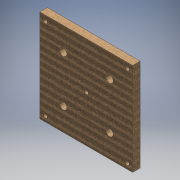
# Autodesk Inventor part: MotorSiliconeMold_1
Saved by Autodesk Inventor 2016 (Build 200138000, 138)
## iProperties
Created: 2015-12-05
Part Number: MotorSiliconeMold_1
Material: MDF Medium Density Fiberboard
Document SubType Name: Modeling
Designer: DonMo
Density: 0.8 g/cm^3
Appearance: Cardboard - Corrugated
BearingDiameter: 24.000 mm
WoodThickness: 6.390 mm
BearingWidth: 7.000 mm
BearingShaftDiameter: 8.000 mm
ZipTieWidth: 2.500 mm
ZipTieThickness: 1.100 mm
ZipTieClearance: 1.000 mm
ZipTieDistance: 10.000 mm
BearingHolderHeight: 13.100 mm
MotorWidth: 37.000 mm
SupportClearance: 5.000 mm
MotorShaftWidth: 12.000 mm
CouplingWidth: 0.375 in
CouplingDiameter: 0.870 in
DiskGap: 75.835 mm
d28: 360.00 deg
SiliconeRingDiameter: 36.224 mm
DowlDiameter: 6.300 mm
HoldScrewDiameter: 3.430 mm
VccumCoverSize: 80.000 mm
Author: DonMo
Autodesk Inventor part; units mm, degrees
ref_plane "YZ Plane" through (0, 0, 0) normal (1, 0, 0) x (0, 1, 0)
ref_plane "XZ Plane" through (0, 0, 0) normal (0, 1, 0) x (-1, 0, 0)
ref_plane "XY Plane" through (0, 0, 0) normal (0, 0, 1) x (1, 0, 0)
sketch "Sketch1" plane through (0, 0, 0) normal (0, 1, 0) x (-1, 0, 0)
  circle A0 centre (20, -20) radius 18.1118 construction
  line L0 (0, 0) -> (80, 0)
  line L1 (80, 0) -> (80, -80)
  line L2 (80, -80) -> (0, -80)
  line L3 (0, -80) -> (0, 0)
  line L4 (40, 0) -> (40, -40) construction
  line L5 (40, -40) -> (80, -40) construction
  line L6 (40, -40) -> (40, -80) construction
  line L7 (40, -40) -> (0, -40) construction
  circle A1 centre (40, -40) radius 1.715
  line L8 (40, -40) -> (0, 0) construction
  circle A2 centre (4.6447, -4.6447) radius 1.715
  circle A3 centre (75.3553, -4.6447) radius 1.715
  circle A4 centre (4.6447, -75.3553) radius 1.715
  circle A5 centre (75.3553, -75.3553) radius 1.715
  circle A6 centre (20, -20) radius 3.15
  circle A7 centre (60, -20) radius 3.15
  circle A8 centre (20, -60) radius 3.15
  circle A9 centre (60, -60) radius 3.15
  point P0 (40, -20)
  point P1 (20, -40)
  dimension "d0" = 36.2235
  dimension "d1" = 80
  dimension "d2" = 80
  dimension "d13" = 3.43
  dimension "d14" = 3.43
  dimension "d15" = 50
  dimension "d16" = 6.3
  constraints: 18 end point, 10 centre point, 6 midpoint, 6 symmetric about line, 3 parallel, 2 coincident, 2 horizontal, 2 horizontal alignment, 1 perpendicular, 1 point on line, 1 vertical alignment, 6 other
  measures "d0" diameter of A0
  measures "d1" distance of L1.end L2.end
  measures "d2" distance of L0.end L1.end
  measures "d13" diameter of A1
  measures "d14" diameter of A2
  measures "d15" distance of L4.end A2.centre
  measures "d16" diameter of A6
extrude "Extrusion3" add sketch "Sketch1" along normal blind 6.39
equation "\"d0\" = SiliconeRingDiameter"
equation "\"d1\" = VccumCoverSize"
equation "\"d2\" = VccumCoverSize"
equation "\"d13\" = HoldScrewDiameter"
equation "\"d14\" = HoldScrewDiameter"
equation "\"d16\" = DowlDiameter"
equation "\"d17\" = WoodThickness"
equation "\"BearingHolderHeight\" = 13.1"
equation "\"SiliconeRingDiameter\" = 0.75 * CouplingDiameter + 1.5 * BearingHolderHeight"
equation "\"DowlDiameter\" = 6.3"
equation "\"HoldScrewDiameter\" = 3.43"
equation "\"VccumCoverSize\" = 80"
equation "\"WoodThickness\" = 6.39"
equation "\"CouplingDiameter\" = 22.098"
body "Solid3"
